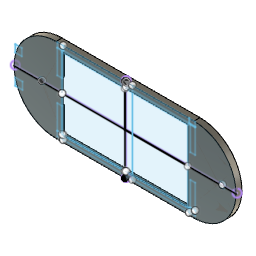
FrontSideSolar_v5 (Autodesk Fusion 360 design; units mm, degrees)
Autodesk Fusion 360 part; units mm, degrees
sketch "Sketch12" plane through (0, 0, 0) normal (0, 1, 0) x (1, 0, 0) in component "Component"
  line L0 (0, 0) -> (115, 0)
  line L1 (115, -70) -> (0, -70)
  arc A0 (0, 0) -> (0, -70) centre (0, -35) ccw
  arc A1 (115, -70) -> (115, 0) centre (115, -35) ccw
  constraint horizontal L0
  constraint horizontal L1
  constraint coincident L0.start A0.start
extrude "Extrude8" add sketch "Sketch12" along normal blind 1 in component "Component"
extrude "Extrude9" add 1 faces at (76.6667, 1, 46.6667) along direction (0, 1, 0) blind 1 thin wall 1 inside in component "Component"
sketch "Sketch13" plane through (0, 1, 0) normal (0, 1, 0) x (-1, 0, 0) in component "Component"
  line L0 (-115, 1) -> (0, 1)
  arc A0 (0, 1) -> (0, 69) centre (0, 35) ccw
  line L1 (0, 69) -> (-115, 69)
  arc A1 (-115, 69) -> (-115, 1) centre (-115, 35) ccw
sketch "Sketch14" plane through (0, 1, 0) normal (0, 1, 0) x (-1, 0, 0) in component "Component"
  circle A0 centre (-137.8811, 35) radius 2.2908
  line L0 (-62.6697, 69.1714) -> (-62.6697, 1)
  circle A1 centre (12.5418, 35) radius 2.2908
  point P0 (12.5418, 35)
  constraint vertical L0
  constraint symmetric A0.centre L0 P0
  constraint symmetric A0 L0 A1
extrude "Extrude10" cut sketch "Sketch14" against normal blind 30 contours A0 in component "Component"
extrude "Extrude11" cut sketch "Sketch14" against normal blind 20 contours A1 in component "Component"
extrude "Extrude12" add 1 faces at (76.6667, 2, 0.3333) along direction (0, 1, 0) blind 1 in component "Component"
extrude "Extrude13" add 1 faces at (76.6667, 3, 0.3333) along direction (0, 1, 0) blind 1 in component "Component"
extrude "Extrude14" add 1 faces at (76.6667, 4, 0.3333) along direction (0, 1, 0) blind 2 in component "Component"
sketch "Sketch15" plane through (0, 1, 0) normal (0, 1, 0) x (-1, 0, 0) in component "Component"
  line L0 (35, 50) -> (29.5357, 50)
  line L1 (29.5357, 50) -> (29.5357, 44)
  line L2 (29.5357, 44) -> (35, 44)
  line L3 (35, 44) -> (35, 50)
  line L4 (35, 20) -> (29, 20)
  line L5 (29, 20) -> (29, 26)
  line L6 (29, 26) -> (35, 26)
  line L7 (35, 26) -> (35, 20)
  dimension "d77" = 6
  dimension "d78" = 6
  constraint horizontal L0
  constraint vertical L1
  constraint horizontal L2
  constraint vertical L3
  constraint horizontal L4
  constraint vertical L5
  constraint horizontal L6
  constraint vertical L7
  measures "d77" distance of L0.start L2.end
  measures "d78" distance of L4.start L6.end
extrude "Extrude15" cut sketch "Sketch15" along normal blind 4 contours L4 L5 L6 L7 in component "Component"
extrude "Extrude16" cut 1 faces at (76.6667, 6, 0.3333) along direction (0, -1, 0) blind 1 in component "Component"
extrude "Extrude17" cut sketch "Sketch15" along normal blind 4 contours L0 L1 L2 L3 in component "Component"
sketch "Sketch16" plane through (0, 0, 0) normal (0, -1, 0) x (1, 0, 0) in component "Component"
  circle A0 centre (-12.5418, 35) radius 2.2908
  circle A1 centre (137.8811, 35) radius 2.2908
  arc A2 (0, 70) -> (0, 0) centre (0, 35) ccw
  line L0 (0, 0) -> (115, 0)
  arc A3 (115, 0) -> (115, 70) centre (115, 35) ccw
  line L1 (115, 70) -> (0, 70)
  line L2 (-35, 35) -> (150, 35)
  line L3 (57.5, 70) -> (57.5, 0)
  line L4 (57.5, 35) -> (110, 35)
  line L5 (110, 35) -> (110, 65)
  line L6 (110, 65) -> (57.5, 65)
  line L7 (57.5, 65) -> (57.5, 35)
  line L8 (5, 65) -> (57.5, 65)
  line L9 (5, 35) -> (5, 65)
  line L10 (5, 35) -> (5, 5)
  line L11 (5, 5) -> (57.5, 5)
  line L12 (110, 5) -> (57.5, 5)
  line L13 (110, 35) -> (110, 5)
  constraint midpoint A2 L2.start
  constraint midpoint A3 L2.end
  constraint coincident L1 L3.start
  constraint coincident L0 L3.end
  constraint perpendicular L0 L3
  constraint symmetric A2 A3 L3
  constraint midpoint L2 L3
  constraint horizontal L4
  constraint vertical L5
  constraint horizontal L6
  constraint vertical L7
  constraint midpoint L3 L4.start
  constraint symmetric L4.end L7 L9.start
  constraint symmetric L5.end L7 L8.start
  constraint symmetric L6.end L7 L8.end
  constraint symmetric L2 L4.end L5.start
  constraint symmetric L2 L5.end L12.start
  constraint symmetric L2 L6.end L11.end
  constraint symmetric L2 L8.start L10.end
  constraint symmetric L2 L9.start L10.start
extrude "Extrude18" cut sketch "Sketch16" against normal blind 1 contours L2 L3 L7 L8 L9 | L2 L3 L10 L11 | L2 L3 L4 L5 L6 L7 | L2 L3 L4 L12 L13 in component "Component"
sketch "Sketch17" plane through (0, 1, 0) normal (0, 1, 0) x (-1, 0, 0) in component "Component"
  line L0 (-111, 65) -> (-115, 65)
  line L1 (-115, 65) -> (-115, 45)
  line L2 (-115, 45) -> (-111, 45)
  line L3 (-111, 45) -> (-111, 65)
  line L4 (35, 35) -> (-150, 35)
  line L5 (-115, 5) -> (-115, 25)
  line L6 (-111, 5) -> (-115, 5)
  line L7 (-111, 25) -> (-111, 5)
  line L8 (-115, 25) -> (-111, 25)
  line L9 (-57.5, 70) -> (-57.5, 0)
  line L10 (0, 65) -> (0, 45)
  line L11 (-4, 45) -> (-4, 65)
  line L12 (-4, 65) -> (0, 65)
  line L13 (0, 45) -> (-4, 45)
  line L14 (0, 25) -> (-4, 25)
  line L15 (0, 5) -> (0, 25)
  line L16 (-4, 25) -> (-4, 5)
  line L17 (-4, 5) -> (0, 5)
  line L18 (-110, 65.5) -> (-57.5, 65.5)
  line L19 (-57.5, 65.5) -> (-57.5, 69)
  line L20 (-57.5, 69) -> (-110, 69)
  line L21 (-110, 69) -> (-110, 65.5)
  line L22 (-5, 65.5) -> (-57.5, 65.5)
  line L23 (-5, 69) -> (-5, 65.5)
  line L24 (-57.5, 65.5) -> (-57.5, 69)
  line L25 (-110, 4.5) -> (-57.5, 4.5)
  line L26 (-57.5, 1) -> (-110, 1)
  line L27 (-110, 1) -> (-110, 4.5)
  line L28 (-57.5, 4.5) -> (-57.5, 1)
  line L29 (-5, 4.5) -> (-57.5, 4.5)
  line L30 (-5, 1) -> (-5, 4.5)
  line L31 (-57.5, 69) -> (-5, 69)
  line L32 (-5, 69) -> (-5, 65.5)
  line L33 (-57.5, 65.5) -> (-57.5, 69)
  line L34 (-57.5, 1) -> (-5, 1)
  line L35 (-57.5, 4.5) -> (-57.5, 1)
  line L36 (-5, 4.5) -> (-57.5, 4.5)
  line L37 (-110, 65.5) -> (-115, 65.5)
  line L38 (-115, 65.5) -> (-115, 69)
  line L39 (-115, 69) -> (-110, 69)
  line L40 (-110, 69) -> (-110, 65.5)
  line L41 (-115, 65.5) -> (-111, 65.5)
  line L42 (-111, 65.5) -> (-111, 65)
  line L43 (-111, 65) -> (-115, 65)
  line L44 (-115, 65) -> (-115, 65.5)
  line L45 (-111, 5) -> (-115, 5)
  line L46 (-115, 4.5) -> (-111, 4.5)
  line L47 (-111, 4.5) -> (-111, 5)
  line L48 (-115, 5) -> (-115, 4.5)
  line L49 (-115, 4.5) -> (-115, 1)
  line L50 (-110, 4.5) -> (-115, 4.5)
  line L51 (-110, 1) -> (-110, 4.5)
  line L52 (-115, 1) -> (-110, 1)
  line L53 (0, 65) -> (-4, 65)
  line L54 (-4, 65) -> (-4, 69)
  line L55 (-4, 69) -> (0, 69)
  line L56 (0, 69) -> (0, 65)
  line L57 (-4, 69) -> (-5, 69)
  line L58 (-5, 69) -> (-5, 65.5)
  line L59 (-5, 65.5) -> (-4, 65.5)
  line L60 (-4, 65.5) -> (-4, 69)
  line L61 (-4, 5) -> (-4, 1)
  line L62 (0, 1) -> (0, 5)
  line L63 (0, 5) -> (-4, 5)
  line L64 (-5, 4.5) -> (-4, 4.5)
  line L65 (-5, 1) -> (-5, 4.5)
  line L66 (-4, 1) -> (-5, 1)
  line L67 (-4, 1) -> (0, 1)
  constraint horizontal L0
  constraint vertical L1
  constraint horizontal L2
  constraint vertical L3
  constraint symmetric L0.start L4 L6.start
  constraint symmetric L0.end L4 L5.start
  constraint symmetric L1.end L4 L5.end
  constraint symmetric L2.end L4 L7.start
  constraint symmetric L0.start L9 L11.end
  constraint symmetric L0.end L9 L10.start
  constraint symmetric L1.end L9 L10.end
  constraint symmetric L2.end L9 L11.start
  constraint symmetric L5.start L9 L15.start
  constraint symmetric L5.end L9 L14.start
  constraint symmetric L6.start L9 L16.end
  constraint symmetric L7.start L9 L14.end
  constraint horizontal L18
  constraint vertical L19
  constraint horizontal L20
  constraint vertical L21
  constraint coincident L9 L19.end
  constraint symmetric L9 L18.start L22.start
  constraint symmetric L9 L18.end L19.start
  constraint symmetric L9 L19.end L20.start
  constraint symmetric L9 L20.end L23.start
  constraint symmetric L4 L18.start L25.start
  constraint symmetric L4 L18.end L25.end
  constraint symmetric L4 L19.end L26.start
  constraint symmetric L4 L20.end L26.end
  constraint symmetric L4 L22.start L29.start
  constraint symmetric L4 L23.start L30.start
  constraint symmetric L9 L25.start L29.start
  constraint symmetric L9 L25.end L28.start
  constraint symmetric L9 L26.start L28.end
  constraint symmetric L9 L26.end L30.start
  constraint horizontal L37
  constraint vertical L38
  constraint horizontal L39
  constraint vertical L40
  constraint horizontal L41
  constraint vertical L42
  constraint horizontal L43
  constraint vertical L44
  constraint symmetric L4 L37.end L46.start
  constraint symmetric L4 L38.end L49.end
  constraint symmetric L4 L41.end L46.end
  constraint symmetric L4 L0.end L5.start
  constraint horizontal L53
  constraint vertical L54
  constraint horizontal L55
  constraint vertical L56
  constraint horizontal L57
  constraint vertical L58
  constraint horizontal L59
  constraint vertical L60
  constraint symmetric L4 L10.start L15.start
  constraint symmetric L4 L11.end L16.end
  constraint symmetric L4 L54.end L61.end
  constraint symmetric L4 L55.end L62.start
  constraint symmetric L4 L59.end L64.end
extrude "Extrude19" add sketch "Sketch17" along normal blind 2 contours L0 L1 L2 L3 L43 | L9 L18 L19 L20 L21 L24 L33 L40 | L9 L19 L22 L23 L24 L31 L32 L33 L58 | L10 L11 L12 L13 L53 | L5 L6 L7 L8 L45 | L9 L25 L26 L27 L28 L35 L51 | L9 L28 L29 L30 L34 L35 L36 L65 | L14 L15 L16 L17 L63 in component "Component"
extrude "Extrude20" add sketch "Sketch17" along normal blind 2 contours L0 L37 L41 L42 L43 L44 | L21 L37 L38 L39 L40 L41 | L23 L32 L54 L57 L58 L59 L60 | L12 L53 L54 L55 L56 L60 | L6 L45 L46 L47 L48 L50 | L27 L46 L49 L50 L51 L52 | L30 L61 L64 L65 L66 | L17 L61 L62 L63 L67 in component "Component"
component "Component" placed x (1, 0, 0) y (0, 1, 0) z (0, 0, 1) at (0, 0, 0)
